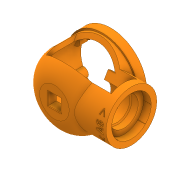
# Autodesk Inventor part: Axis 6 Gearbox
Saved by Autodesk Inventor 2020 (Build 240168000, 168)
## iProperties
Created: 2021-06-29
Part Number: Axis 6 Gearbox
Material: Generic
Document SubType Name: Modeling
Designer: Coy
Density: 1 g/cm^3
Appearance: Orange
Author: Coy
Autodesk Inventor part; units mm, degrees
ref_plane "XZ Plane" through (0, 0, 0) normal (0, 1, 0) x (-1, 0, 0)
ref_plane "XY Plane" through (0, 0, 0) normal (0, 0, 1) x (1, 0, 0)
sketch "Sketch1" plane through (0, 0, 0) normal (0, 0, 1) x (1, 0, 0)
  circle A0 centre (0, 0) radius 6
  dimension "d0" = 12
  constraints: 1 centre point, 1 coincident
  measures "d0" diameter of A0
extrude "Extrusion1" add sketch "Sketch1" against normal blind 8
chamfer "Chamfer1" distance 8 angle 2 1 edges at (-6, 0, -8) measured on face at (-6, 0, -7.5)
sketch "Sketch2" plane through (0, 0, -8) normal (0, 0, -1) x (-1, 0, 0)
  circle A0 centre (0, 0) radius 6 construction
  circle A1 centre (0, 0) radius 5.7206 projected
  line L0 (0, 0) -> (0, 8.298) construction
  arc A2 (0.1999, 5.9933) -> (-0.1999, 5.9933) centre (0, 6) ccw
  line L1 (0.1907, 5.7175) -> (0.2, 5.9967)
  line L2 (-0.1907, 5.7175) -> (-0.2, 5.9967)
  arc A3 (-5.0904, 3.1698) -> (-5.2903, 2.8236) centre (-5.1962, 3) ccw
  line L3 (-5.0468, 2.6936) -> (-5.2933, 2.8251)
  line L4 (-4.8561, 3.0239) -> (-5.0933, 3.1715)
  arc A4 (-5.2903, -2.8236) -> (-5.0904, -3.1698) centre (-5.1962, -3) ccw
  line L5 (-4.8561, -3.0239) -> (-5.0933, -3.1715)
  line L6 (-5.0468, -2.6936) -> (-5.2933, -2.8251)
  arc A5 (-0.1999, -5.9933) -> (0.1999, -5.9933) centre (0, -6) ccw
  line L7 (0.1907, -5.7175) -> (0.2, -5.9967)
  line L8 (-0.1907, -5.7175) -> (-0.2, -5.9967)
  arc A6 (5.0904, -3.1698) -> (5.2903, -2.8236) centre (5.1962, -3) ccw
  line L9 (5.0468, -2.6936) -> (5.2933, -2.8251)
  line L10 (4.8561, -3.0239) -> (5.0933, -3.1715)
  arc A7 (5.2903, 2.8236) -> (5.0904, 3.1698) centre (5.1962, 3) ccw
  line L11 (4.8561, 3.0239) -> (5.0933, 3.1715)
  line L12 (5.0468, 2.6936) -> (5.2933, 2.8251)
  dimension "d6" = 0.4
  dimension "d9" = 360
  constraints: 26 end point, 17 point on circle, 13 point on line, 6 centre point, 2 line through centre, 2 tangent, 1 vertical, 61 other
  measures "d6" diameter of A2
extrude "Extrusion2" add sketch "Sketch2" against normal up to surface (8 mm away) contours A1 L11 A7 L12 | L9 A6 L10 A1 | A1 L2 A2 L1 | L7 A5 L8 A1 | A1 L3 A3 L4 | L5 A4 L6 A1
sketch "Sketch3" plane through (0, 0, 0) normal (0, 0, 1) x (1, 0, 0)
  arc A0 (-0.2, 5.9967) -> (-5.0933, 3.1715) centre (0, 0) ccw projected
  arc A1 (-5.0933, 3.1715) -> (-5.2933, 2.8252) centre (-5.1962, 3) ccw projected
  arc A2 (-5.2933, 2.8252) -> (-5.2933, -2.8252) centre (0, 0) ccw projected
  arc A3 (-5.2933, -2.8252) -> (-5.0933, -3.1715) centre (-5.1962, -3) ccw projected
  arc A4 (-5.0933, -3.1715) -> (-0.2, -5.9967) centre (0, 0) ccw projected
  arc A5 (-0.2, -5.9967) -> (0.2, -5.9967) centre (0, -6) ccw projected
  arc A6 (0.2, -5.9967) -> (5.0933, -3.1715) centre (0, 0) ccw projected
  arc A7 (5.0933, -3.1715) -> (5.2933, -2.8252) centre (5.1962, -3) ccw projected
  arc A8 (5.2933, -2.8252) -> (5.2933, 2.8252) centre (0, 0) ccw projected
  arc A9 (5.2933, 2.8252) -> (5.0933, 3.1715) centre (5.1962, 3) ccw projected
  arc A10 (5.0933, 3.1715) -> (0.2, 5.9967) centre (0, 0) ccw projected
  arc A11 (0.2, 5.9967) -> (-0.2, 5.9967) centre (0, 6) ccw projected
extrude "Extrusion3" add sketch "Sketch3" along normal blind 0.5
sketch "Sketch4" plane through (0, 0, 0.5) normal (0, 0, 1) x (1, 0, 0)
  circle A0 centre (0, 0) radius 32.5
  dimension "d15" = 65
  constraints: 1 centre point, 1 coincident
  measures "d15" diameter of A0
extrude "Extrusion4" add sketch "Sketch4" along normal blind 4
sketch "Sketch5" plane through (0, 0, 4.5) normal (0, 0, 1) x (1, 0, 0)
  circle A0 centre (0, 0) radius 32.5
  circle A1 centre (0, 0) radius 28.5
  dimension "d18" = 4
  constraints: 2 centre point, 1 coincident
  measures "d18" radial gap between concentric circles of A0 A1
extrude "Extrusion5" add sketch "Sketch5" along normal blind 32
sketch "Sketch6" plane through (0, 0, 0) normal (1, 0, 0) x (0, 1, 0)
  line L0 (2.6936, -8) -> (-2.6936, -8) construction
  line L1 (0, -8) -> (0, 93.9815)
  line L2 (-14, 58) -> (14, 58)
  line L3 (32.5, 36.5) -> (-32.5, 36.5) projected
  line L4 (32.5, 0.5) -> (32.5, 36.5) construction
  line L5 (-32.5, 0.5) -> (-32.5, 36.5) construction
  arc A0 (32.5, 36.5) -> (14, 58) centre (10.7568, 36.5) ccw
  arc A1 (28.5, 36.5) -> (13.6847, 54) centre (10.7568, 36.5) ccw
  line L6 (13.6847, 54) -> (-14, 54)
  line L7 (14, 58) -> (14, 40.3088)
  point P0 (0, 0)
  point P1 (0, 58)
  point P2 (0, 54)
  point P3 (14, 53.9443)
  dimension "d21" = 28
  dimension "d22" = 14
  dimension "d23" = 21.5
  dimension "d24" = 4
  constraints: 8 end point, 4 point on circle, 3 vertical, 2 centre point, 1 horizontal, 1 midpoint, 1 tangent, 1 other
  measures "d21" distance of L2.start L2.end
  measures "d22" distance from line of L1 L2.end
  measures "d23" distance between parallel lines of L3 L2
  measures "d24" radial gap between concentric circles of A0 A1
revolve "Revolution1" add sketch "Sketch6" angle 360 about axis through (0, 0, -8) along (0, 0, 1) contours A1 L7 A0 L3
ref_plane "Work Plane1" through (0, 0, 54) normal (0, 0, -1) x (-1, 0, 0)
sketch "Sketch7" plane through (0, 0, 54) normal (0, 0, -1) x (-1, 0, 0)
  circle A0 centre (0, 0) radius 14 projected
  circle A1 centre (0, 0) radius 18
  point P0 (0, 0)
  dimension "d27" = 4
  constraints: 1 centre point
  measures "d27" radial gap between concentric circles of A0 A1
extrude "Extrusion6" add sketch "Sketch7" along normal blind 4
ref_plane "Work Plane2" through (0, 0, 58) normal (0, 0, -1) x (-1, 0, 0)
ref_plane "Work Plane3" through (48, 0, 0) normal (1, 0, 0) x (0, 1, 0)
sketch "Sketch9" plane through (48, 0, 0) normal (1, 0, 0) x (0, 1, 0)
  line L0 (32.5, 0.5) -> (-32.5, 0.5) construction
  line L1 (47.8895, 33) -> (-46.9798, 33) construction
  line L2 (0, 0) -> (0, 66.4464) construction
  circle A0 centre (0, 33) radius 24
  circle A1 centre (0, 33) radius 18.5
  dimension "d42" = 32.5
  dimension "d43" = 48
  dimension "d44" = 5.5
  constraints: 4 end point, 2 centre point, 2 point on line, 1 horizontal, 1 vertical
  measures "d42" distance between parallel lines of L0 L1
  measures "d43" diameter of A0
  measures "d44" radial gap between concentric circles of A0 A1
extrude "Extrusion8" add sketch "Sketch9" against normal up to next
sketch "Sketch10" plane through (48, 0, 33) normal (1, 0, 0) x (0, 0, -1)
  circle A0 centre (0, 0) radius 18.5 projected
  point P0 (33, 0)
extrude "Extrusion9" cut sketch "Sketch10" against normal blind 30
chamfer "Chamfer3" distance 7 angle 2 2 edges at (48, -13.0815, 46.0815) (48, 13.0815, 19.9185) measured on face at (47.5, 13.0815, 19.9185) measured on face at (47.5, -13.0815, 46.0815)
sketch "Sketch11" plane through (48, 0, 33) normal (1, 0, 0) x (0, 0, -1)
  circle A0 centre (0, 0) radius 18.5 construction
  circle A1 centre (0, 0) radius 18.7444 projected
  line L0 (0, 0) -> (0, 37.3695) construction
  arc A2 (-0.2, 18.4989) -> (0.2, 18.4989) centre (0, 18.5) ccw
  line L1 (0.2026, 18.7433) -> (0.2, 18.4978)
  line L2 (-0.2026, 18.7433) -> (-0.2, 18.4978)
  line L3 (-13.3968, 13.1103) -> (-13.2214, 12.9385)
  arc A3 (-13.2221, 12.9393) -> (-12.9393, 13.2221) centre (-13.0815, 13.0815) ccw
  line L4 (-13.1103, 13.3968) -> (-12.9385, 13.2214)
  line L5 (-18.7433, -0.2026) -> (-18.4978, -0.2)
  arc A4 (-18.4989, -0.2) -> (-18.4989, 0.2) centre (-18.5, 0) ccw
  line L6 (-18.7433, 0.2026) -> (-18.4978, 0.2)
  line L7 (-13.1103, -13.3968) -> (-12.9385, -13.2214)
  arc A5 (-12.9393, -13.2221) -> (-13.2221, -12.9393) centre (-13.0815, -13.0815) ccw
  line L8 (-13.3968, -13.1103) -> (-13.2214, -12.9385)
  line L9 (0.2026, -18.7433) -> (0.2, -18.4978)
  arc A6 (0.2, -18.4989) -> (-0.2, -18.4989) centre (0, -18.5) ccw
  line L10 (-0.2026, -18.7433) -> (-0.2, -18.4978)
  line L11 (13.3968, -13.1103) -> (13.2214, -12.9385)
  arc A7 (13.2221, -12.9393) -> (12.9393, -13.2221) centre (13.0815, -13.0815) ccw
  line L12 (13.1103, -13.3968) -> (12.9385, -13.2214)
  line L13 (18.7433, 0.2026) -> (18.4978, 0.2)
  arc A8 (18.4989, 0.2) -> (18.4989, -0.2) centre (18.5, 0) ccw
  line L14 (18.7433, -0.2026) -> (18.4978, -0.2)
  line L15 (13.1103, 13.3968) -> (12.9385, 13.2214)
  arc A9 (12.9393, 13.2221) -> (13.2221, 12.9393) centre (13.0815, 13.0815) ccw
  line L16 (13.3968, 13.1103) -> (13.2214, 12.9385)
  point P0 (33, 0)
  point P1 (14.2828, 14)
  point P2 (13.3968, 13.1103)
  point P3 (13.1103, 13.3968)
  point P4 (19.999, -0.2)
  point P5 (18.7433, -0.2026)
  point P6 (18.7433, 0.2026)
  point P7 (14, -14.2828)
  point P8 (13.1103, -13.3968)
  point P9 (13.3968, -13.1103)
  point P10 (-0.2, -19.999)
  point P11 (0.2026, -18.7433)
  point P12 (-14.2828, -14)
  point P13 (-13.1103, -13.3968)
  point P14 (-19.999, 0.2)
  point P15 (-18.7433, 0.2026)
  point P16 (-18.7433, -0.2026)
  point P17 (-14, 14.2828)
  point P18 (-13.1103, 13.3968)
  point P19 (-13.3968, 13.1103)
  point P20 (-0.2, 19.999)
  point P21 (0.2, 19.999)
  point P22 (12.9393, 13.2221)
  point P23 (13.2221, 12.9393)
  point P24 (18.4989, 0.2)
  point P25 (18.4989, -0.2)
  point P26 (13.2221, -12.9393)
  point P27 (12.9393, -13.2221)
  point P28 (0.2, -18.4989)
  point P29 (-0.2, -18.4989)
  point P30 (-12.9393, -13.2221)
  point P31 (-13.2221, -12.9393)
  point P32 (-18.4989, -0.2)
  point P33 (-18.4989, 0.2)
  point P34 (-13.2221, 12.9393)
  point P35 (-12.9393, 13.2221)
  point P36 (-0.2, 18.4989)
  point P37 (0.2, 18.4989)
  dimension "d52" = 0.4
  dimension "d55" = 360
  constraints: 37 point on circle, 34 end point, 8 centre point, 2 line through centre, 2 tangent, 1 point on line, 1 vertical, 81 other
  measures "d52" diameter of A2
extrude "Extrusion10" add sketch "Sketch11" against normal blind 7 contours A1 L14 A8 L13 | L16 A9 L15 A1 | A1 L12 A7 L11 | L4 A3 L3 A1 | A1 L8 A5 L7 | L6 A4 L5 A1
ref_plane "Work Plane4" through (41, 0, 33) normal (1, 0, 0) x (0, 0, -1)
sketch "Sketch12" plane through (41, 0, 33) normal (1, 0, 0) x (0, 0, -1)
  arc A0 (12.9393, 13.2221) -> (-12.9393, 13.2221) centre (0, 0) ccw projected
  circle A1 centre (0, 0) radius 20
  circle A2 centre (0, 0) radius 12.5
  point P0 (33, 0)
  point P1 (-0.2, 18.4989)
  point P2 (-56, 57.1314)
  point P3 (-0.8, 79.996)
  dimension "d166" = 25
  constraints: 2 centre point, 2 coincident, 1 other
  measures "d166" diameter of A2
extrude "Extrusion11" add sketch "Sketch12" against normal blind 25
sketch "Sketch13" plane through (0, 0, 50) normal (0, 0, -1) x (-1, 0, 0)
  circle A0 centre (0, 0) radius 14 projected
  circle A1 centre (0, 0) radius 6.05
  point P0 (0, 0)
  dimension "d63" = 12.1
  constraints: 1 centre point, 1 coincident
  measures "d63" diameter of A1
extrude "Extrusion12" add sketch "Sketch13" against normal blind 8
sketch "Sketch14" plane through (0, 0, 58) normal (0, 0, 1) x (1, 0, 0)
  circle A0 centre (0, 0) radius 6.05 construction
  circle A1 centre (0, 0) radius 4.05
  line L0 (0, 0) -> (0, 10.1919) construction
  line L1 (-6.1, 6.1) -> (6.1, 6.1)
  line L2 (6.1, 6.1) -> (6.1, -6.1)
  line L3 (6.1, -6.1) -> (-6.1, -6.1)
  line L4 (-6.1, -6.1) -> (-6.1, 6.1)
  line L5 (0, 0) -> (0, 13.5563)
  line L6 (0, 0) -> (-13.2473, 0)
  point P0 (0, 0)
  point P1 (0.6694, 3.9943)
  point P2 (-0.6694, 3.9943)
  dimension "d66" = 2
  dimension "d253" = 12.2
  dimension "d254" = 12.2
  constraints: 14 end point, 2 horizontal, 2 parallel, 2 point on circle, 2 vertical, 1 centre point, 1 perpendicular, 2 other
  measures "d66" radial gap between concentric circles of A0 A1
  measures "d253" distance of L2.end L3.end
  measures "d254" distance of L1.end L2.end
extrude "Extrusion13" cut sketch "Sketch14" against normal blind 8 contours A1 L5 L1 L2 L3 L4 L6 | A1 L6 L4 L1 L5
ref_plane "Work Plane5" through (41, 0, 33) normal (1, 0, 0) x (0, 0, -1)
sketch "Sketch16" plane through (41, 0, 33) normal (1, 0, 0) x (0, 0, -1)
  line L0 (0, 0) -> (-21.7229, 37.6252)
  line L1 (0, 0) -> (22.5437, 39.0468)
  line L2 (0, 0) -> (12.9488, 0) construction
  line L3 (22.5437, 39.0468) -> (-21.7229, 37.6252)
  circle A0 centre (0, 0) radius 12.5 projected
  point P0 (33, 0)
  point P1 (-6.25, 10.8253)
  point P2 (6.25, 10.8253)
  dimension "d172" = 60
  dimension "d173" = 60
  dimension "d174" = 0
  dimension "d175" = 0
  constraints: 8 end point, 1 coincident, 1 horizontal
  measures "d172" angle of L1 L0
  measures "d173" angle of L2 L1
  measures "d174" distance from line of point (0, 0) L2
  measures "d175" distance of point (0, 0) L0.start
extrude "Extrusion15" cut sketch "Sketch16" against normal blind 60 contours L0 L3 L1 A0
sketch "Sketch17" plane through (16, 0, 33) normal (-1, 0, 0) x (0, 0, 1)
  arc A0 (-6.25, 10.8253) -> (6.25, 10.8253) centre (0, 0) ccw projected
  line L0 (0, 0) -> (42.5553, 0) construction
  circle A1 centre (5.25, 0) radius 4
  arc A2 (5.25, 6) -> (1.0074, -4.2426) centre (5.25, 0) ccw
  line L1 (5.25, 6) -> (17, 6)
  line L2 (3.5, 21.2426) -> (3.5, -28.5) projected
  line L3 (1.0074, -4.2426) -> (12.4317, -15.667)
  line L4 (17, 8.2462) -> (17, -8.2462) projected
  line L5 (-6.25, 10.8253) -> (-10, 17.3205) projected
  arc A3 (-10, 17.3205) -> (18.2209, -8.2462) centre (0, 0) ccw projected
  line L6 (17, -8.2462) -> (18.2209, -8.2462) projected
  line L7 (17, 8.2462) -> (17, -8.2462) projected
  line L8 (18.2209, 8.2462) -> (17, 8.2462) projected
  arc A4 (18.2209, 8.2462) -> (10, 17.3205) centre (0, 0) ccw projected
  line L9 (10, 17.3205) -> (6.25, 10.8253) projected
  arc A5 (-6.25, 10.8253) -> (6.25, 10.8253) centre (0, 0) ccw projected
  line L10 (17, -8.2462) -> (17, -10.5357)
  line L11 (17, 18) -> (17, -18) projected
  line L12 (17, -8.2462) -> (-4.2491, -8.2462)
  point P0 (-33, 0)
  point P1 (3.5, -19.6914)
  point P2 (5.0109, -8.2462)
  point P3 (17, 6)
  dimension "d178" = 8
  dimension "d179" = 5.25
  dimension "d180" = 2
  dimension "d181" = 45
  constraints: 10 end point, 4 point on circle, 3 point on line, 2 centre point, 2 perpendicular, 2 tangent, 1 horizontal
  measures "d178" diameter of A1
  measures "d179" distance of L0.start A1.centre
  measures "d180" radial gap between concentric circles of A1 A2
  measures "d181" angle of L0 L3
extrude "Extrusion16" add sketch "Sketch17" along normal blind 5 contours L12 L3 L2 A1 A2 L1 A0 | A0 L1 L4 L12 | L3 A2 L2 A1
ref_plane "Work Plane6" through (23.5, 0, 33) normal (-1, 0, 0) x (0, 0, -1)
sketch "Sketch19" plane through (23.5, 0, 33) normal (-1, 0, 0) x (0, 0, -1)
  line L0 (-1.0074, 4.2426) -> (-5.0109, 8.2462) projected
  arc A0 (-5.25, -6) -> (-1.0074, 4.2426) centre (-5.25, 0) ccw projected
  line L1 (-17, -6) -> (-5.25, -6) projected
  arc A1 (-6.25, -10.8253) -> (6.25, -10.8253) centre (0, 0) ccw projected
  line L2 (-5.0109, 8.2462) -> (-17, 8.2462) projected
  line L3 (-17, -6) -> (-17, 8.2462) projected
  line L4 (-5.0109, 8.2462) -> (-8.868, 12.1033)
  arc A2 (6.25, -10.8253) -> (-9.3941, 8.2462) centre (0, 0) ccw projected
  arc A3 (-7.0719, 10.3072) -> (-9.3941, 8.2462) centre (0, 0) ccw
  point P0 (33, 0)
  point P1 (-7.0719, -10.3072)
  point P2 (-10.9659, 6)
  constraints: 3 point on circle, 2 end point, 1 centre point, 1 point on line
extrude "Extrusion18" add sketch "Sketch19" against normal blind 5
sketch "Sketch21" plane through (28.5, 0, 33) normal (1, 0, 0) x (0, 0, -1)
  arc A0 (-1.0074, -4.2426) -> (-5.25, 6) centre (-5.25, 0) ccw projected
  circle A1 centre (-5.25, 0) radius 4
  point P0 (33, 0)
  dimension "d193" = 8
  constraints: 1 centre point, 1 coincident
  measures "d193" diameter of A1
extrude "Extrusion20" cut sketch "Sketch21" against normal blind 2.5
sketch "Sketch22" plane through (26, 0, 38.25) normal (1, 0, 0) x (0, 0, -1)
  circle A0 centre (0, 0) radius 4 projected
  circle A1 centre (0, 0) radius 3
  point P0 (38.25, 0)
  dimension "d196" = 6
  constraints: 1 centre point, 1 coincident
  measures "d196" diameter of A1
extrude "Extrusion21" cut sketch "Sketch22" against normal blind 2.5 contours A1
sketch "Sketch23" plane through (16, 0, 33) normal (1, 0, 0) x (0, 0, -1)
  circle A0 centre (-5.25, 0) radius 3 projected
  circle A1 centre (-5.25, 0) radius 4 projected
  point P0 (33, 0)
extrude "Extrusion22" add sketch "Sketch23" against normal blind 2.5
chamfer "Chamfer34" distance 1.5 angle 2 1 edges at (11, 0, 34.25) measured on face at (11.5, 0, 34.25)
chamfer "Chamfer35" distance 1.5 angle 2 1 edges at (28.5, 0, 42.25) measured on face at (28, 0, 42.25)
fillet "Fillet1" radius 0.5 2 edges at (28.5, 0, 42.3024) (11, 0, 34.1976)
ref_plane "Work Plane7" through (48, 0, 57) normal (0, 0, 1) x (1, 0, 0)
sketch "Sketch24" plane through (48, 0, 57) normal (0, 0, 1) x (1, 0, 0)
  line L0 (-11.7043, -23.6043) -> (-11.7043, 23.766) construction
  line L1 (-11.7043, 23.766) -> (-0.0638, 23.766) construction
  line L2 (-0.0638, 23.766) -> (-0.0638, -23.6043) construction
  line L3 (-0.0638, -23.6043) -> (-11.7043, -23.6043) construction
  line L4 (-2.9028, -8.7791) -> (-5.0863, -14.0353)
  line L5 (-5.0863, -14.0353) -> (-5.9854, -14.0353)
  line L6 (-5.9854, -14.0353) -> (-8.1689, -8.7791)
  line L7 (-8.1689, -8.7791) -> (-7.0376, -8.7791)
  line L8 (-7.0376, -8.7791) -> (-5.5309, -12.4545)
  line L9 (-5.5309, -12.4545) -> (-4.034, -8.7791)
  line L10 (-4.034, -8.7791) -> (-2.9028, -8.7791)
  line L11 (-2.8435, -5.4841) -> (-8.9395, -3.4241)
  line L12 (-8.9395, -3.4241) -> (-8.9395, -1.7544)
  line L13 (-8.9395, -1.7544) -> (-2.8435, 0.3056)
  line L14 (-2.8435, 0.3056) -> (-2.8435, -1.2703)
  line L15 (-2.8435, -1.2703) -> (-4.0884, -1.6506)
  line L16 (-4.0884, -1.6506) -> (-4.0884, -3.5674)
  line L17 (-4.0884, -3.5674) -> (-2.8435, -3.9527)
  line L18 (-2.8435, -3.9527) -> (-2.8435, -5.4841)
  line L19 (-5.195, -1.9866) -> (-7.2105, -2.609)
  line L20 (-7.2105, -2.609) -> (-5.195, -3.2364)
  line L21 (-5.195, -3.2364) -> (-5.195, -1.9866)
  spline S0 degree 2 poles (-4.9183, 5.3444) (-3.955, 5.3444) (-2.7151, 4.1243) (-2.7151, 3.0572) knots 0 0 0 1 2 2 2
  spline S1 degree 2 poles (-2.7151, 3.0572) (-2.7151, 2.5237) (-3.0213, 1.6888) (-3.3227, 1.3974) knots 0 0 0 1 2 2 2
  spline S2 degree 2 poles (-3.3227, 1.3974) (-3.6734, 1.0516) (-4.7849, 0.6811) (-5.5605, 0.6811) knots 0 0 0 1 2 2 2
  spline S3 degree 2 poles (-5.5605, 0.6811) (-6.3608, 0.6811) (-7.6057, 1.0269) (-8.0849, 1.4171) knots 0 0 0 1 2 2 2
  spline S4 degree 2 poles (-8.0849, 1.4171) (-8.5394, 1.7876) (-9.0531, 2.993) (-9.0531, 3.818) knots 0 0 0 1 2 2 2
  spline S5 degree 2 poles (-9.0531, 3.818) (-9.0531, 4.1193) (-8.9741, 4.722) (-8.9494, 4.8307) knots 0 0 0 1 2 2 2
  line L22 (-8.9494, 4.8307) -> (-7.7539, 4.8307)
  line L23 (-7.7539, 4.8307) -> (-7.7539, 4.722)
  spline S6 degree 2 poles (-7.7539, 4.722) (-7.8082, 4.6133) (-7.9416, 4.1193) (-7.9416, 3.8032) knots 0 0 0 1 2 2 2
  spline S7 degree 2 poles (-7.9416, 3.8032) (-7.9416, 3.0868) (-7.1858, 2.3063) (-6.4843, 2.2125) knots 0 0 0 1 2 2 2
  spline S8 degree 2 poles (-6.4843, 2.2125) (-6.677, 2.5138) (-6.9042, 3.1313) (-6.9042, 3.5216) knots 0 0 0 1 2 2 2
  spline S9 degree 2 poles (-6.9042, 3.5216) (-6.9042, 3.8526) (-6.7264, 4.4305) (-6.5584, 4.6528) knots 0 0 0 1 2 2 2
  spline S10 degree 2 poles (-6.5584, 4.6528) (-6.3163, 4.969) (-5.5309, 5.3444) (-4.9183, 5.3444) knots 0 0 0 1 2 2 2
  spline S11 degree 2 poles (-3.9995, 3.5611) (-4.1477, 3.6797) (-4.4935, 3.8081) (-4.8442, 3.8081) knots 0 0 0 1 2 2 2
  spline S12 degree 2 poles (-4.8442, 3.8081) (-5.1406, 3.8081) (-5.5259, 3.6599) (-5.6396, 3.5265) knots 0 0 0 1 2 2 2
  spline S13 degree 2 poles (-5.6396, 3.5265) (-5.7581, 3.3882) (-5.8421, 3.0473) (-5.8421, 2.8547) knots 0 0 0 1 2 2 2
  spline S14 degree 2 poles (-5.8421, 2.8547) (-5.8421, 2.6916) (-5.7581, 2.3557) (-5.6988, 2.2075) knots 0 0 0 1 2 2 2
  spline S15 degree 2 poles (-5.6988, 2.2075) (-5.6593, 2.2075) (-5.4716, 2.1976) (-5.3283, 2.1976) knots 0 0 0 1 2 2 2
  spline S16 degree 2 poles (-5.3283, 2.1976) (-4.7997, 2.1976) (-4.1625, 2.3804) (-3.9995, 2.5237) knots 0 0 0 1 2 2 2
  spline S17 degree 2 poles (-3.9995, 2.5237) (-3.8661, 2.6274) (-3.7525, 2.9041) (-3.7525, 3.0523) knots 0 0 0 1 2 2 2
  spline S18 degree 2 poles (-3.7525, 3.0523) (-3.7525, 3.1758) (-3.876, 3.4623) (-3.9995, 3.5611) knots 0 0 0 1 2 2 2
  line L24 (-5.0863, 14.197) -> (-2.9028, 8.9408)
  line L25 (-2.9028, 8.9408) -> (-4.034, 8.9408)
  line L26 (-4.034, 8.9408) -> (-5.5358, 12.6112)
  line L27 (-5.5358, 12.6112) -> (-7.0376, 8.9408)
  line L28 (-7.0376, 8.9408) -> (-8.1689, 8.9408)
  line L29 (-8.1689, 8.9408) -> (-5.9854, 14.197)
  line L30 (-5.9854, 14.197) -> (-5.0863, 14.197)
  point P0 (-48, 0)
  constraints: 2 other
emboss "Emboss1" sketch "Sketch24" operation cut depth 1 direction (0, 0, -1) wrap yes faces at (38.0029, -0.132, 56.9996)
chamfer "Chamfer36" distance 2 angle 45 3 edges at (16, -1.3707, 45.4246) (23.5, -9.3491, 41.2973) (23.5, -1.3707, 45.4246)
sketch "Sketch25" plane through (0, 0, 0.5) normal (0, 0, -1) x (-1, 0, 0)
  arc A0 (0.2, -5.9967) -> (5.0933, -3.1715) centre (0, 0) ccw construction
  circle A1 centre (0, 0) radius 27 construction
  circle A2 centre (0, 0) radius 32.5 construction
  dimension "d214" = 54
  constraints: 1 centre point, 1 coincident
  measures "d214" diameter of A1
ref_plane "Work Plane8" through (0, 0, 4.5) normal (0, 0, -1) x (-1, 0, 0)
sketch "Sketch28" plane through (0, 0, -8) normal (0, 0, -1) x (-1, 0, 0)
  circle A0 centre (0, 0) radius 32.5 construction
  circle A1 centre (0, 0) radius 32.5 projected
extrude "Extrusion23" cut sketch "Sketch28" against normal blind 12.5
sketch "Sketch29" plane through (0, 0, 4.5) normal (0, 0, -1) x (-1, 0, 0)
  line L0 (0, 0) -> (45.0441, 0) construction
  circle A0 centre (0, 0) radius 32.5
  circle A1 centre (0, 0) radius 29.75 construction
  circle A2 centre (29.75, 0) radius 2 construction
  circle A3 centre (25.7643, 14.875) radius 2 construction
  circle A4 centre (14.875, 25.7643) radius 2 construction
  circle A5 centre (0, 29.75) radius 2 construction
  circle A6 centre (-14.875, 25.7643) radius 2 construction
  circle A7 centre (-25.7643, 14.875) radius 2 construction
  circle A8 centre (-29.75, 0) radius 2 construction
  circle A9 centre (-25.7643, -14.875) radius 2 construction
  circle A10 centre (-14.875, -25.7643) radius 2 construction
  circle A11 centre (0, -29.75) radius 2 construction
  circle A12 centre (14.875, -25.7643) radius 2 construction
  circle A13 centre (25.7643, -14.875) radius 2 construction
  circle A14 centre (0, 29.75) radius 2.5
  circle A15 centre (-14.875, 25.7643) radius 2.5
  circle A16 centre (14.875, 25.7643) radius 2.5
  circle A17 centre (25.7643, 14.875) radius 2.5
  circle A18 centre (-25.7643, 14.875) radius 2.5
  circle A19 centre (-25.7643, -14.875) radius 2.5
  circle A20 centre (-14.875, -25.7643) radius 2.5
  circle A21 centre (0, -29.75) radius 2.5
  circle A22 centre (14.875, -25.7643) radius 2.5
  circle A23 centre (25.7643, -14.875) radius 2.5
  arc A24 (-29.8196, 12.9245) -> (-26.1027, 19.3623) centre (-25.7643, 14.875) ccw
  arc A25 (-19.3623, 26.1027) -> (-12.9245, 29.8196) centre (-14.875, 25.7643) ccw
  arc A26 (-3.7168, 32.2868) -> (3.7168, 32.2868) centre (0, 29.75) ccw
  arc A27 (12.9245, 29.8196) -> (19.3623, 26.1027) centre (14.875, 25.7643) ccw
  arc A28 (26.1027, 19.3623) -> (29.8196, 12.9245) centre (25.7643, 14.875) ccw
  arc A29 (29.8196, -12.9245) -> (26.1027, -19.3623) centre (25.7643, -14.875) ccw
  arc A30 (19.3623, -26.1027) -> (12.9245, -29.8196) centre (14.875, -25.7643) ccw
  arc A31 (3.7168, -32.2868) -> (-3.7168, -32.2868) centre (0, -29.75) ccw
  arc A32 (-12.9245, -29.8196) -> (-19.3623, -26.1027) centre (-14.875, -25.7643) ccw
  arc A33 (-26.1027, -19.3623) -> (-29.8196, -12.9245) centre (-25.7643, -14.875) ccw
  dimension "d221" = 2.75
  dimension "d222" = 4
  dimension "d223" = 360
  dimension "d224" = 5
  dimension "d225" = 5
  dimension "d226" = 5
  dimension "d227" = 5
  dimension "d228" = 5
  dimension "d229" = 5
  dimension "d230" = 5
  dimension "d231" = 5
  dimension "d232" = 5
  dimension "d233" = 5
  dimension "d234" = 2
  dimension "d235" = 2
  dimension "d236" = 2
  dimension "d237" = 2
  dimension "d238" = 2
  dimension "d239" = 2
  dimension "d240" = 2
  dimension "d241" = 2
  dimension "d242" = 2
  dimension "d243" = 2
  constraints: 32 centre point, 20 point on circle, 10 coincident, 2 end point, 1 horizontal, 1 horizontal alignment, 1 point on line, 49 other
  measures "d222" diameter of A2
  measures "d224" diameter of A14
  measures "d225" diameter of A15
  measures "d226" diameter of A16
  measures "d227" diameter of A17
  measures "d228" diameter of A18
  measures "d229" diameter of A19
  measures "d230" diameter of A20
  measures "d231" diameter of A21
  measures "d232" diameter of A22
  measures "d233" diameter of A23
  measures "d234" radial gap between concentric circles of A18 A24
  measures "d235" radial gap between concentric circles of A15 A25
  measures "d236" radial gap between concentric circles of A14 A26
  measures "d237" radial gap between concentric circles of A16 A27
  measures "d238" radial gap between concentric circles of A17 A28
  measures "d239" radial gap between concentric circles of A23 A29
  measures "d240" radial gap between concentric circles of A22 A30
  measures "d241" radial gap between concentric circles of A21 A31
  measures "d242" radial gap between concentric circles of A20 A32
  measures "d243" radial gap between concentric circles of A19 A33
extrude "Extrusion24" add sketch "Sketch29" against normal blind 8 contours A28 A0 | A0 A29 | A27 A0 | A0 A30 | A26 A0 | A0 A31 | A25 A0 | A0 A32 | A24 A0 | A0 A33
sketch "Sketch30" plane through (0, 0, 4.5) normal (0, 0, -1) x (-1, 0, 0)
  arc A0 (-25.6723, 12.3767) -> (-23.5547, 16.0445) centre (-25.7643, 14.875) ccw construction
  arc A1 (-16.0445, 23.5547) -> (-12.3767, 25.6723) centre (-14.875, 25.7643) ccw construction
  arc A2 (-2.1176, 28.4212) -> (2.1176, 28.4212) centre (0, 29.75) ccw construction
  arc A3 (12.3767, 25.6723) -> (16.0445, 23.5547) centre (14.875, 25.7643) ccw construction
  arc A4 (23.5547, 16.0445) -> (25.6723, 12.3767) centre (25.7643, 14.875) ccw construction
  arc A5 (-23.5547, -16.0445) -> (-25.6723, -12.3767) centre (-25.7643, -14.875) ccw construction
  arc A6 (-12.3767, -25.6723) -> (-16.0445, -23.5547) centre (-14.875, -25.7643) ccw construction
  line L0 (19, 21.2426) -> (19, 18.9805) construction
  arc A7 (-17.6633, -3.4655) -> (-17.6633, 3.4655) centre (0, 0) ccw construction
  arc A8 (-20.6034, -19.6914) -> (19, 21.2426) centre (0, 0) ccw construction
  arc A9 (2.1176, -28.4212) -> (-2.1176, -28.4212) centre (0, -29.75) ccw construction
  circle A10 centre (0, 0) radius 27 construction
  arc A11 (25.6723, -12.3767) -> (23.5547, -16.0445) centre (25.7643, -14.875) ccw construction
  arc A12 (16.0445, -23.5547) -> (12.3767, -25.6723) centre (14.875, -25.7643) ccw construction
  circle A13 centre (-14.875, 25.7643) radius 2.5
  circle A14 centre (0, 29.75) radius 2.5
  arc A15 (12.3767, 25.6723) -> (16.0445, 23.5547) centre (14.875, 25.7643) ccw projected
  circle A16 centre (14.875, 25.7643) radius 2.5
  circle A17 centre (25.7643, 14.875) radius 2.5
  circle A18 centre (25.7643, -14.875) radius 2.5
  circle A19 centre (14.875, -25.7643) radius 2.5
  circle A20 centre (0, -29.75) radius 2.5
  circle A21 centre (-14.875, -25.7643) radius 2.5
  circle A22 centre (-25.7643, -14.875) radius 2.5
  circle A23 centre (-25.7643, 14.875) radius 2.5
  point P0 (12.3767, 25.6723)
  constraints: 10 coincident, 8 centre point, 6 concentric, 9 other
extrude "Extrusion25" cut sketch "Sketch30" against normal blind 8
sketch "Sketch31" plane through (0, 0, 4.5) normal (0, 0, -1) x (-1, 0, 0)
  circle A0 centre (0, 0) radius 32.5 projected
  circle A1 centre (0, 0) radius 34
  dimension "d248" = 1.5
  constraints: 1 centre point
  measures "d248" radial gap between concentric circles of A0 A1
extrude "Extrusion26" add sketch "Sketch31" against normal blind 8
sketch "Sketch32" plane through (0, 0, 12.5) normal (0, 0, 1) x (1, 0, 0)
  arc A0 (10.4388, 26.5194) -> (17.7471, 22.3) centre (14.875, 25.7643) ccw projected
  arc A1 (-4.2194, 28.1859) -> (4.2194, 28.1859) centre (0, 29.75) ccw projected
  arc A2 (-17.7471, 22.3) -> (-10.4388, 26.5194) centre (-14.875, 25.7643) ccw projected
  arc A3 (-26.5194, 10.4388) -> (-22.3, 17.7471) centre (-25.7643, 14.875) ccw projected
  arc A4 (22.3, 17.7471) -> (26.5194, 10.4388) centre (25.7643, 14.875) ccw projected
  arc A5 (26.5194, -10.4388) -> (22.3, -17.7471) centre (25.7643, -14.875) ccw projected
  arc A6 (17.7471, -22.3) -> (10.4388, -26.5194) centre (14.875, -25.7643) ccw projected
  arc A7 (4.2194, -28.1859) -> (-4.2194, -28.1859) centre (0, -29.75) ccw projected
  arc A8 (-10.4388, -26.5194) -> (-17.7471, -22.3) centre (-14.875, -25.7643) ccw projected
  arc A9 (-22.3, -17.7471) -> (-26.5194, -10.4388) centre (-25.7643, -14.875) ccw projected
  arc A10 (-26.5194, 10.4388) -> (-26.5194, -10.4388) centre (0, 0) ccw projected
  circle A11 centre (0, 0) radius 28.5
  circle A12 centre (0, 0) radius 34
  point P0 (-4.2194, 28.1859)
  point P1 (4.2194, 28.1859)
  point P2 (10.4388, 26.5194)
  point P3 (17.7471, 22.3)
  point P4 (22.3, 17.7471)
  point P5 (26.5194, 10.4388)
  point P6 (26.5194, -10.4388)
  point P7 (17.7471, -22.3)
  point P8 (10.4388, -26.5194)
  point P9 (4.2194, -28.1859)
  point P10 (-4.2194, -28.1859)
  point P11 (-10.4388, -26.5194)
  point P12 (-17.7471, -22.3)
  point P13 (-22.3, -17.7471)
  point P14 (-22.3, 17.7471)
  point P15 (-17.7471, 22.3)
  point P16 (-10.4388, 26.5194)
  constraints: 2 coincident, 1 centre point, 3 other
extrude "Extrusion27" add sketch "Sketch32" against normal blind 1 contours A11 A0 | A1 A11 | A11 A4 | A2 A11 | A11 A5 | A3 A11 | A11 A6 | A9 A11 | A11 A7 | A8 A11 | A12
fillet "Fillet3" radius 0.5 4 edges at (0, 6.1, 58) (-6.1, 0, 58) (0, -6.1, 58) (6.1, 0, 58)
sketch "Sketch34" plane through (41, 0, 33) normal (1, 0, 0) x (0, 0, -1)
  arc A0 (-6.25, 10.8253) -> (6.25, 10.8253) centre (0, 0) ccw projected
  arc A1 (-6.75, 11.6913) -> (6.75, 11.6913) centre (0, 0) ccw
  line L0 (9.25, 16.0215) -> (6.25, 10.8253) projected
  line L1 (-6.25, 10.8253) -> (-9.25, 16.0215) projected
  point P0 (33, 0)
  dimension "d258" = 1
  constraints: 2 point on circle, 1 centre point
  measures "d258" radial gap between concentric circles of A0 A1
extrude "Extrusion29" cut sketch "Sketch34" against normal blind 6
chamfer "Chamfer37" distance 1 angle 45 2 edges at (35, 6.25, 22.1747) (35, -10.8253, 39.25)
sketch "Sketch35" plane through (-25.7643, 14.875, 11.5) normal (0, 0, -1) x (-1, 0, 0)
  circle A0 centre (-51.5285, 0) radius 2.5 projected
  circle A1 centre (-40.6393, 10.8893) radius 2.5 projected
  circle A2 centre (-25.7643, 14.875) radius 2.5 projected
  circle A3 centre (-10.8893, 10.8893) radius 2.5 projected
  circle A4 centre (0, 0) radius 2.5 projected
  circle A5 centre (0, -29.75) radius 2.5 projected
  circle A6 centre (-10.8893, -40.6393) radius 2.5 projected
  circle A7 centre (-25.7643, -44.625) radius 2.5 projected
  circle A8 centre (-40.6393, -40.6393) radius 2.5 projected
  circle A9 centre (-51.5285, -29.75) radius 2.5 projected
  point P0 (-25.7643, -14.875)
extrude "Extrusion30" add sketch "Sketch35" along normal blind 3
equation "\"d22\" = 0.5 * d21"
equation "\"d61\" = d166"
body "Solid1"
